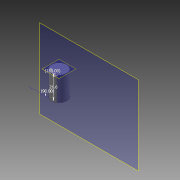
# Autodesk Inventor part: MOTOR
Saved by Autodesk Inventor 2014 (Build 180170000, 170)
## iProperties
Created: 2013-09-20
Part Number: MOTOR
Material: Generic
Document SubType Name: Modeling
Designer: Brandon
Density: 1 g/cm^3
Appearance: Default
Author: Brandon
Autodesk Inventor part; units mm, degrees
ref_plane "YZ Plane" through (0, 0, 0) normal (1, 0, 0) x (0, 1, 0)
ref_plane "XZ Plane" through (0, 0, 0) normal (0, 1, 0) x (-1, 0, 0)
ref_plane "XY Plane" through (0, 0, 0) normal (0, 0, 1) x (1, 0, 0)
sketch "Sketch1" plane through (0, 0, 0) normal (0, 0, 1) x (1, 0, 0)
  circle A0 centre (0, 0) radius 8.5
  circle A1 centre (0, 0) radius 3.075
  circle A2 centre (0, 0) radius 0.75
  line L0 (0, 0) -> (-3.6062, -3.6062) construction
  line L1 (0, 0) -> (5.1, 0) construction
  line L2 (0, 0) -> (3.6062, 3.6062) construction
  line L3 (0, 0) -> (5.1, 0) construction
  circle A3 centre (-3.6062, -3.6062) radius 1
  circle A4 centre (3.6216, 3.6216) radius 1
  dimension "d0" = 17
  dimension "d1" = 6.15
  dimension "d2" = 1.5
  dimension "d3" = 5.1
  dimension "d4" = 135
  dimension "d5" = 5.1
  dimension "d6" = 45
  dimension "d7" = 2
  dimension "d8" = 2
  constraints: 8 end point, 5 centre point, 4 coincident, 2 equal length, 2 horizontal, 1 collinear
  measures "d0" diameter of A0
  measures "d1" diameter of A1
  measures "d2" diameter of A2
  measures "d3" distance of L0.start L0.end
  measures "d4" angle of L0 L1
  measures "d5" distance of L0.start L2.end
  measures "d6" angle of L3 L2
  measures "d7" diameter of A3
  measures "d8" diameter of A4
extrude "Extrusion1" add sketch "Sketch1" along normal blind 3 contours A0 | A1 | A2
ref_plane "Work Plane1" through (-7.1967, -146.8933, 23.5) normal (1, 0, 0) x (0, 1, 0)
sketch "Sketch2" plane through (-7.1967, -146.8933, 23.5) normal (1, 0, 0) x (0, 1, 0)
  line L0 (146.8933, -23.5) -> (146.8933, 3.1)
  line L1 (146.8933, -23.5) -> (173.4933, -23.5) construction
  line L2 (146.8933, 3.1) -> (141.8933, 3.1)
  line L3 (146.8933, 3.1) -> (151.8933, 3.1) construction
  dimension "d11" = 26.6
  dimension "d12" = 90
  dimension "d13" = 5
  dimension "d14" = 180
  constraints: 8 end point, 2 equal length, 2 horizontal, 1 parallel, 1 vertical
  measures "d11" distance of L0.start L0.end
  measures "d12" angle of L1 L0
  measures "d13" distance of L0.end L2.end
  measures "d14" angle of L2 L3
ref_plane "Work Plane4" through (0, 0, 26.6) normal (0, 0, -1) x (-1, 0, 0)
extrude "Extrusion2" add sketch "Sketch1" along normal up to surface (23.6 mm away) from surface at 3 contours A0 | A1 | A2 | A3 | A4
extrude "Extrusion3" add sketch "Sketch1" against normal blind 1.65 contours A1 | A2
extrude "Extrusion4" add sketch "Sketch1" against normal blind 4.05 contours A2
equation "\"d5\" = d3"
equation "\"d8\" = d7"
body "Solid1"
